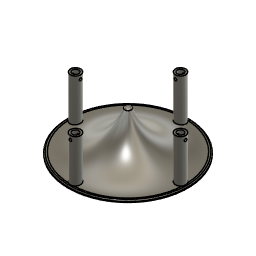
Speaker Stand (Autodesk Fusion 360 design; units mm, degrees)
Autodesk Fusion 360 part; units mm, degrees
note: some values were not read from the file. Set by a fixed rule: which sketch regions a step uses.
sketch "base" plane through (0, 0, 0) normal (0, 1, 0) x (1, 0, 0)
  circle A0 centre (0, 0) radius 46
  circle A1 centre (0, 0) radius 44
  dimension "d1" = 92
  dimension "d2" = 88
  constraint coincident A0.centre A1.centre
  measures "d1" diameter of A0
  measures "d2" diameter of A1
sketch "cone" plane through (0, 0, 0) normal (1, 0, 0) x (0, 0, -1)
  line L0 (0, 0) -> (0, 30)
  circle A0 through (44, 0, 0) (-22, 0, 38.1051) (-22, 0, -38.1051) construction
  line L1 (0, 0, 0) -> (-44, 0, -0.0077)
  line L2 (0, 0) -> (-2.5, 0) construction
  line L3 (-2.5, 0) -> (-2.5, 29) construction
  arc A1 through (-44, 0, -0.0077) (-18.6857, 7.9684, -0.0032) (-2.5, 29, -0.0004)
  arc A2 (0, 30) -> (-2.5, 29) centre (-0.8012, 28.378) ccw
  dimension "d3" = 30
  dimension "d6" = 2.5
  dimension "d7" = 29
  constraint coincident L0.start L2.start
  constraint vertical L0
  constraint perpendicular L0 L2
  constraint perpendicular L2 L3
  measures "d3" distance of L0.start L0.end
  measures "d6" distance of L0.start L2.end
  measures "d7" distance of L2.end L3.end
extrude "Extrude1" add sketch "base" against normal blind 1.5 contours A0 | A1
sketch "cone (curves on the plane with normal 1, 0, 0.0002 at 0 mm)" plane through (0, 0, 0) normal (1, 0, 0.000174) x (0, -1, 0)
  line L0 (0, 0) -> (-30, 0)
  line L1 (0, 0) -> (0, -44)
  line L2 (0, 0) -> (0, -2.5) construction
  line L3 (0, -2.5) -> (-29, -2.5) construction
  arc A0 (0, -44) -> (-29, -2.5) centre (-44.194, -44) ccw
  arc A1 (-30, 0) -> (-29, -2.5) centre (-28.378, -0.8012) ccw
revolve "Revolve1" add sketch "cone (curves on the plane with normal 1, 0, 0.0002 at 0 mm)" angle 360 about axis through (0, 0, 0) along (0, 1, 0)
sketch "posts" plane through (0, 0, 0) normal (0, 1, 0) x (1, 0, 0)
  circle A0 centre (0, 0) radius 40.5 construction
  circle A1 centre (40.5, 0) radius 2.5
  circle A2 centre (40.5, 0) radius 4
  circle A3 centre (0, 40.5) radius 4
  circle A4 centre (0, 40.5) radius 2.5
  circle A5 centre (-40.5, 0) radius 4
  circle A6 centre (-40.5, 0) radius 2.5
  circle A7 centre (0, -40.5) radius 4
  circle A8 centre (0, -40.5) radius 2.5
  dimension "d9" = 81
  dimension "d10" = 5
  dimension "d11" = 8
  dimension "d12" = 8
  dimension "d13" = 5
  dimension "d14" = 8
  dimension "d15" = 5
  dimension "d16" = 8
  dimension "d17" = 5
  constraint coincident A0.centre origin
  constraint coincident A0 A1.centre
  constraint concentric A1 A2
  constraint coincident A0 A3.centre
  constraint concentric A3 A4
  constraint coincident A0 A5.centre
  constraint concentric A5 A6
  constraint coincident A0 A7.centre
  constraint concentric A7 A8
  measures "d9" diameter of A0
  measures "d10" diameter of A1
  measures "d11" diameter of A2
  measures "d12" diameter of A3
  measures "d13" diameter of A4
  measures "d14" diameter of A5
  measures "d15" diameter of A6
  measures "d16" diameter of A7
  measures "d17" diameter of A8
extrude "Extrude2" add sketch "posts" along normal blind 33 contours A1 | A2 | A3 | A4 | A5 | A6 | A7 | A8
extrude "Extrude3" cut sketch "posts" along normal blind 6 from surface at 27 contours A1 | A4 | A6 | A8
sketch "filament" plane through (0, 0, 0) normal (0, 0, 1) x (1, 0, 0)
  line L0 (0, 0, -40.5) -> (0, 30, -40.5) construction
  circle A0 through (1, 30, -40.5) (-0.5, 30.866, -40.5) (-0.5, 29.134, -40.5)
  line L1 (40.5, 0) -> (40.5, 30) construction
  line L2 (0, 0, 40.5) -> (0, 30, 40.5) construction
  line L3 (-40.5, 0) -> (-40.5, 30) construction
  circle A1 through (1, 30, 40.5) (-0.5, 30.866, 40.5) (-0.5, 29.134, 40.5)
  circle A2 through (40.5, 31, 0) (40.5, 29.5, 0.866) (40.5, 29.5, -0.866)
  circle A3 through (-40.5, 31, 0) (-40.5, 29.5, 0.866) (-40.5, 29.5, -0.866)
  point P0 (40.5, 0)
  point P1 (-40.5, 0)
  dimension "d23" = 30
  dimension "d24" = 2
  dimension "d25" = 30
  dimension "d26" = 30
  dimension "d27" = 30
  dimension "d28" = 2
  dimension "d47" = 2
  dimension "d48" = 2
  constraint coincident P0 L1.start
  constraint vertical L1
  constraint coincident P1 L3.start
  measures "d25" distance of P0 L1.end
  measures "d27" distance of P1 L3.end
sketch "filament (curves -40.5 mm off its plane)" plane through (0, 0, -40.5) normal (0, 0, 1) x (1, 0, 0)
  line L0 (0, 0) -> (0, 30) construction
  circle A0 centre (0, 30) radius 1
extrude "Extrude4" cut sketch "filament (curves -40.5 mm off its plane)" along normal blind 4 and the other way blind 4
sketch "filament (curves 40.5 mm off its plane)" plane through (0, 0, 40.5) normal (0, 0, 1) x (1, 0, 0)
  line L0 (0, 0) -> (0, 30) construction
  circle A0 centre (0, 30) radius 1
extrude "Extrude6" cut sketch "filament (curves 40.5 mm off its plane)" along normal blind 4 and the other way blind 4
sketch "filament (curves on the plane with normal 1, 0, 0 at -40.5 mm)" plane through (-40.5, 0, 0) normal (1, 0, 0) x (0, 1, 0)
  line L0 (0, 0) -> (30, 0) construction
  circle A0 centre (30, 0) radius 1
extrude "Extrude8" cut sketch "filament (curves on the plane with normal 1, 0, 0 at -40.5 mm)" against normal blind 4 and the other way blind 4
sketch "filament (curves on the plane with normal 1, 0, 0 at 40.5 mm)" plane through (40.5, 0, 0) normal (1, 0, 0) x (0, 1, 0)
  line L0 (0, 0) -> (30, 0) construction
  circle A0 centre (30, 0) radius 1
extrude "Extrude9" cut sketch "filament (curves on the plane with normal 1, 0, 0 at 40.5 mm)" against normal blind 4 and the other way blind 4
fillet "Fillet1" radius 0.75 1 edges at (-42.8871, 0, 16.6343)
equation "d3 = ConeHeight"
equation "d7 = ConeHeight - ConeOffset"
equation "d9 = MountRing"
equation "d10 = InnerSupport"
equation "d11 = OuterSupport"
equation "d12 = OuterSupport"
equation "d13 = InnerSupport"
equation "d14 = OuterSupport"
equation "d15 = InnerSupport"
equation "d16 = OuterSupport"
equation "d17 = InnerSupport"
equation "d18 = SupportHeight"
equation "d20 = SupportHeight - PostHeight"
equation "d21 = PostHeight"
equation "d23 = SupportHeight - HoleHeight"
equation "d24 = Filament"
equation "d25 = SupportHeight - HoleHeight"
equation "d26 = SupportHeight - HoleHeight"
equation "d27 = SupportHeight - HoleHeight"
equation "d28 = Filament"
equation "d31 = HoleLength"
equation "d33 = HoleLength"
equation "d39 = HoleLength"
equation "d41 = HoleLength"
equation "d47 = Filament"
equation "d48 = Filament"
equation "d49 = HoleLength"
equation "d51 = HoleLength"
equation "d53 = HoleLength"
equation "d55 = HoleLength"
equation "InnerSupport = 5 mm"
equation "OuterSupport = 8 mm"
equation "Post = 4.5 mm"
equation "Filament = 2 mm"
equation "HoleLength = 4 mm"
equation "SupportHeight = ConeHeight + 3 mm"
equation "PostHeight = 6 mm"
equation "HoleHeight = 3 mm"
equation "ConeHeight = 30 mm"
equation "ConeOffset = 1 mm"
equation "MountRing = 81 mm"
named bodies: "Speaker Stand"
